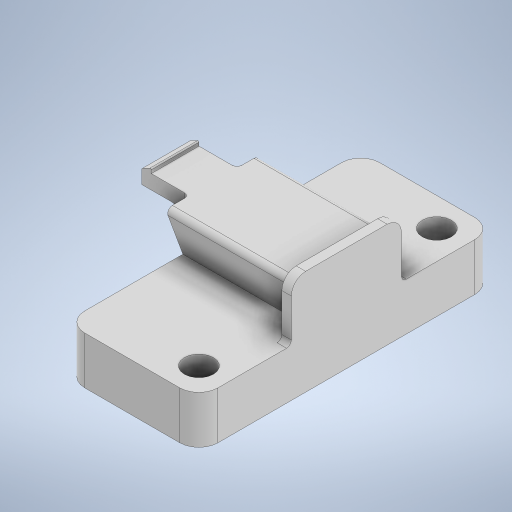
# Autodesk Inventor part: male1
Saved by Autodesk Inventor 2023 (Build 270158000, 158)
## iProperties
Created: 2024-01-15
Part Number: male1
Material: Generic
Document SubType Name: Modeling
Designer: User
Density: 1 g/cm^3
Appearance: Default
Author: User
Autodesk Inventor part; units mm, degrees
ref_plane "YZ Plane" through (0, 0, 0) normal (1, 0, 0) x (0, 1, 0)
ref_plane "XZ Plane" through (0, 0, 0) normal (0, 1, 0) x (-1, 0, 0)
ref_plane "XY Plane" through (0, 0, 0) normal (0, 0, 1) x (1, 0, 0)
sketch "Sketch1" plane through (0, 0, 0) normal (0, 1, 0) x (-1, 0, 0)
  line L0 (-1, -15.5) -> (1, -15.5)
  line L1 (1, 15.5) -> (-1, 15.5)
  line L2 (-3, 13.5) -> (-3, -13.5)
  line L3 (-3, -15.5) -> (3, 15.5) construction
  line L4 (3, -15.5) -> (-3, 15.5) construction
  circle A0 centre (0, 12.5) radius 1.525
  circle A1 centre (0, -12.5) radius 1.525
  arc A2 (-1, 15.5) -> (-3, 13.5) centre (-1, 13.5) ccw
  arc A3 (-3, -13.5) -> (-1, -15.5) centre (-1, -13.5) ccw
  line L5 (1, -15.5) -> (9, -15.5)
  line L6 (11, -13.5) -> (11, 13.5)
  line L7 (9, 15.5) -> (1, 15.5)
  arc A4 (9, -15.5) -> (11, -13.5) centre (9, -13.5) ccw
  arc A5 (11, 13.5) -> (9, 15.5) centre (9, 13.5) ccw
  point P0 (0, 0)
  point P1 (11, -15.5)
  dimension "d0" = 25
  dimension "d1" = 3.05
  dimension "d2" = 3.05
  dimension "d3" = 3
  dimension "d4" = 3
  dimension "d7" = 31
  dimension "d19" = 10
  dimension "d20" = 2
  constraints: 16 end point, 8 point on circle, 8 point on line, 8 tangent, 6 centre point, 2 horizontal, 2 midpoint, 2 perpendicular, 1 equal radius, 1 parallel
  measures "d0" distance of A1.centre A0.centre
  measures "d1" diameter of A1
  measures "d2" diameter of A0
  measures "d3" distance from line of A0.centre L1
  measures "d4" distance from line of L0 A1.centre
  measures "d7" distance between parallel lines of L1 L0
  measures "d19" distance of L0.end point (11, -15.5)
  measures "d20" radius of A4
extrude "Extrusion1" add sketch "Sketch1" along normal blind 5
sketch "Sketch2" plane through (3, 0, 13.5) normal (1, 0, 0) x (0, 0, -1)
  line L0 (0, 5) -> (27, 5) projected
  line L1 (27, 5) -> (0, 5) projected
  line L2 (13.5, 5) -> (13.5, 10)
  line L3 (13.5, 10) -> (17.7859, 10)
  line L4 (18.2558, 9.329) -> (16.6801, 5)
  line L5 (13.5, 10) -> (9.2141, 10)
  line L6 (8.7442, 9.329) -> (10.3199, 5)
  line L7 (10.3199, 5) -> (16.6801, 5)
  arc A0 (9.2141, 10) -> (8.7442, 9.329) centre (9.2141, 9.5) ccw
  arc A1 (18.2558, 9.329) -> (17.7859, 10) centre (17.7859, 9.5) ccw
  point P0 (13.5, 0)
  point P1 (18.5, 10)
  point P2 (8.5, 10)
  dimension "d11" = 5
  dimension "d12" = 5
  dimension "d13" = 70
  dimension "d14" = 5
  dimension "d15" = 70
  dimension "d16" = 0.5
  constraints: 12 end point, 6 point on line, 4 point on circle, 4 tangent, 2 centre point, 1 collinear, 1 equal radius, 1 horizontal, 1 midpoint, 1 perpendicular, 1 vertical
  measures "d11" distance of L2.start L2.end
  measures "d12" distance of L2.end point (18.5, 10)
  measures "d13" angle of L3 L4
  measures "d14" distance of L2.end point (8.5, 10)
  measures "d15" angle of L6 L5
  measures "d16" radius of A0
extrude "Extrusion2" add sketch "Sketch2" against normal up to surface (14 mm away)
sketch "Sketch3" plane through (3, 10, 4.2859) normal (0, 1, 0) x (1, 0, 0)
  line L0 (-14, 8.5719) -> (-14, 0) projected
  line L1 (-14, 1.7859) -> (-19, 1.7859)
  line L2 (-19, 1.7859) -> (-19, 6.7859)
  line L3 (-19, 6.7859) -> (-14, 6.7859)
  line L4 (-14, 6.7859) -> (-14, 1.7859)
  line L5 (0, 8.5719) -> (-14, 8.5719) projected
  point P0 (-3, 4.2859)
  point P1 (-14, 4.2859)
  point P2 (-14, 6.7859)
  dimension "d21" = 5
  dimension "d22" = 5
  constraints: 8 end point, 2 midpoint, 2 parallel, 1 horizontal, 1 perpendicular, 1 point on line
  measures "d21" distance of L2.end L3.end
  measures "d22" distance of L1.end L2.end
extrude "Extrusion3" add sketch "Sketch3" against normal blind 1.5
sketch "Sketch4" plane through (-11, 10, -2.5) normal (0, 0, -1) x (-1, 0, 0)
  line L0 (5, 0) -> (0, 0) projected
  line L1 (5, 0) -> (4, 0)
  line L2 (4, 0) -> (4, 0.3382)
  line L3 (4.1447, 0.4276) -> (5, 0)
  arc A0 (4.1447, 0.4276) -> (4, 0.3382) centre (4.1, 0.3382) ccw
  point P0 (-11, -10)
  point P1 (4, 0.5)
  dimension "d26" = 1
  dimension "d27" = 0.5
  dimension "d28" = 0.1
  constraints: 6 end point, 3 point on line, 2 point on circle, 2 tangent, 1 centre point, 1 perpendicular
  measures "d26" distance of L0.start L1.end
  measures "d27" distance of L1.end point (4, 0.5)
  measures "d28" radius of A0
extrude "Extrusion4" add sketch "Sketch4" against normal up to surface (5 mm away)
fillet "Fillet1" radius 2 1 edges at (-11, 8.5, 0)
fillet "Fillet2" radius 0.2 1 edges at (-16, 10, 0)
sketch "Sketch5" plane through (3, 0, 13.5) normal (1, 0, 0) x (0, 0, -1)
  line L0 (0, 0) -> (27, 0) projected
  line L1 (27, 0) -> (27, 5) projected
  line L2 (16.6801, 5) -> (27, 5) projected
  line L3 (16.6801, 5) -> (18.2558, 9.329) projected
  arc A0 (18.2558, 9.329) -> (17.7859, 10) centre (17.7859, 9.5) ccw projected
  line L4 (17.7859, 10) -> (9.2141, 10) projected
  arc A1 (9.2141, 10) -> (8.7442, 9.329) centre (9.2141, 9.5) ccw projected
  line L5 (8.7442, 9.329) -> (10.3199, 5) projected
  line L6 (0, 5) -> (10.3199, 5) projected
  line L7 (0, 0) -> (0, 5) projected
  line L8 (9.2141, 11) -> (17.7859, 11)
  arc A2 (19.2859, 9.5) -> (17.7859, 11) centre (17.7859, 9.5) ccw
  arc A3 (9.2141, 11) -> (7.7141, 9.5) centre (9.2141, 9.5) ccw
  line L9 (7.7141, 9.5) -> (7.7141, 5)
  line L10 (19.2859, 9.5) -> (19.2859, 5)
  line L11 (7.7141, 5) -> (19.2859, 5)
  point P0 (13.5, 0)
  dimension "d33" = 1
  constraints: 8 end point, 4 point on circle, 2 centre point, 2 perpendicular, 2 point on line, 1 horizontal, 1 tangent
  measures "d33" distance between parallel lines of L4 L8
extrude "Extrusion5" add sketch "Sketch5" against normal blind 1 contours L9 A3 L8 A2 L10 L2 L3 A0 L4 A1 L5 L6
fillet "Fillet3" radius 0.5 1 edges at (2.5, 5, 5.7859)
fillet "Fillet4" radius 0.5 3 edges at (2.5, 5, -5.7859) (-11, 8.25, 2.5) (-11, 8.25, -2.5)
equation "\"d2\" = d1"
equation "\"d4\" = d3"
body "Solid1"
